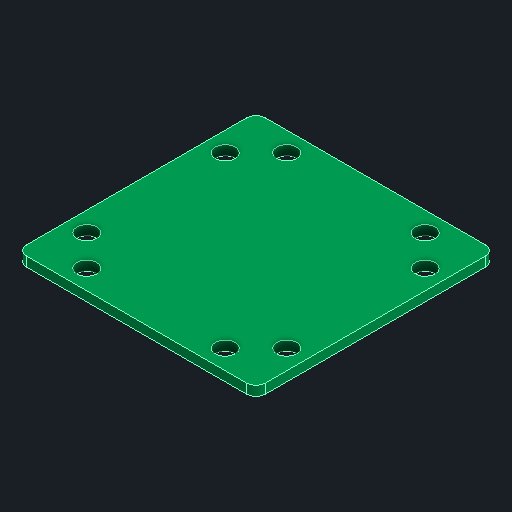
# Autodesk Inventor part: Outer Cover Top
Saved by Autodesk Inventor 2023.4 (Build 274418000, 418)
## iProperties
Created: 2024-07-23
Part Number: Outer Cover Top
Material: Generic
Document SubType Name: Modeling
Designer: xSibe
Density: 1 g/cm^3
Appearance: Plastic Dark Green
Author: xSibe
Autodesk Inventor part; units mm, degrees
ref_plane "YZ Plane" through (0, 0, 0) normal (1, 0, 0) x (0, 1, 0)
ref_plane "XZ Plane" through (0, 0, 0) normal (0, 1, 0) x (-1, 0, 0)
ref_plane "XY Plane" through (0, 0, 0) normal (0, 0, 1) x (1, 0, 0)
sketch "Sketch1" plane through (0, 0, 0) normal (0, 1, 0) x (-1, 0, 0)
  line L0 (-155.225, -15) -> (-155.225, 15) projected
  line L1 (-155.225, 15) -> (-147.725, 15) projected
  line L2 (-147.725, 15) -> (-147.725, -15) projected
  line L3 (-147.725, -15) -> (-155.225, -15) projected
  circle A0 centre (-171.5, -21.9) radius 1.875 projected
  circle A1 centre (-127.7, 21.9) radius 1.875 projected
  circle A2 centre (-127.7, -21.9) radius 1.875 projected
  circle A3 centre (-171.5, 21.9) radius 1.875 projected
  circle A4 centre (-135.2, 20.8) radius 2.0734 projected
  circle A5 centre (-164, -20.8) radius 2.0734 projected
  circle A6 centre (-135.2, -20.8) radius 2.0734 projected
  circle A7 centre (-128.8, -14.4) radius 2.0734 projected
  circle A8 centre (-128.8, 14.4) radius 2.0734 projected
  circle A9 centre (-164, 20.8) radius 2.0734 projected
  circle A10 centre (-170.4, -14.4) radius 2.0734 projected
  circle A11 centre (-170.4, 14.4) radius 2.0734 projected
  line L4 (-172.5, 24.875) -> (-126.7, 24.875) projected
  arc A12 (-172.5, 24.875) -> (-174.475, 22.9) centre (-172.5, 22.9) ccw projected
  line L5 (-174.475, -22.9) -> (-174.475, 22.9) projected
  arc A13 (-174.475, -22.9) -> (-172.5, -24.875) centre (-172.5, -22.9) ccw projected
  line L6 (-126.7, -24.875) -> (-172.5, -24.875) projected
  arc A14 (-126.7, -24.875) -> (-124.725, -22.9) centre (-126.7, -22.9) ccw projected
  line L7 (-124.725, 22.9) -> (-124.725, -22.9) projected
  arc A15 (-124.725, 22.9) -> (-126.7, 24.875) centre (-126.7, 22.9) ccw projected
  point P0 (0, 0)
ref_plane "Work Plane1" through (124.725, 49.8, -24.875) normal (0, 1, 0) x (0, 0, 1)
extrude "Extrusion1" add sketch "Sketch1" along normal blind 2 from surface at 49.8 contours L0 L1 L2 L3 | A0 | A1 | A2 | A3 | L4 A15 L7 A14 L6 A13 L5 A12
body "Solid1"
